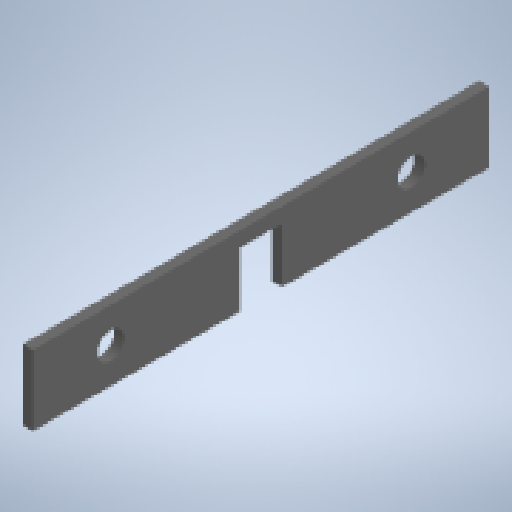
# Autodesk Inventor part: battery_holder_cover
Saved by Autodesk Inventor 2024.1 (Build 281209000, 209)
## iProperties
Created: 2025-03-06
Part Number: battery_holder_cover
Material: 一般
Document SubType Name: Modeling
Designer: hibik
Density: 1 g/cm^3
Appearance: 既定
Author: hibik
Autodesk Inventor part; units mm, degrees
ref_plane "YZ Plane" through (0, 0, 0) normal (1, 0, 0) x (0, 1, 0)
ref_plane "XZ Plane" through (0, 0, 0) normal (0, 1, 0) x (-1, 0, 0)
ref_plane "XY Plane" through (0, 0, 0) normal (0, 0, 1) x (1, 0, 0)
sketch "スケッチ1" plane through (0, 0, 0) normal (1, 0, 0) x (0, 1, 0)
  line L0 (0, 0) -> (7, 0)
  line L1 (7, 0) -> (7, -45.5)
  line L2 (7, -45.5) -> (0, -45.5)
  line L3 (0, -45.5) -> (0, 0)
  line L4 (0, -20.65) -> (5.5, -20.65)
  line L5 (5.5, -20.65) -> (5.5, -24.85)
  line L6 (5.5, -24.85) -> (0, -24.85)
  line L7 (0, -24.85) -> (0, -20.65)
  point P0 (5.5, -22.75)
  point P1 (0, -22.75)
  dimension "d0" = 45.5
  dimension "d1" = 7
  dimension "d2" = 4.2
  dimension "d3" = 1.5
  constraints: 16 end point, 4 parallel, 2 horizontal, 2 midpoint, 2 perpendicular, 1 horizontal alignment, 1 point on line
  measures "d0" distance of L0.end L1.end
  measures "d1" distance of L1.end L2.end
  measures "d2" distance of L4.end L5.end
  measures "d3" distance between parallel lines of L1 L5
extrude "押し出し1" add sketch "スケッチ1" along normal blind 1 contours L0 L1 L2 L3 L6 L5 L4
sketch "スケッチ2" plane through (0, 0, 0) normal (-1, 0, 0) x (0, 0, 1)
  circle A0 centre (-37.75, 3.5) radius 1.6
  circle A1 centre (-7.75, 3.5) radius 1.6
  line L0 (-45.5, 7) -> (0, 7) projected
  line L1 (-45.5, 7) -> (0, 7) projected
  line L2 (-22.75, 7) -> (-22.75, 0)
  line L3 (0, 0) -> (-20.65, 0) projected
  point P0 (-22.75, 3.5)
  dimension "d6" = 3.2
  dimension "d8" = 30
  constraints: 2 centre point, 2 end point, 2 midpoint, 1 equal radius, 1 horizontal alignment, 1 point on line, 1 symmetric about line, 1 vertical
  measures "d6" diameter of A0
  measures "d8" distance of A1.centre A0.centre
extrude "押し出し2" cut sketch "スケッチ2" against normal through all
